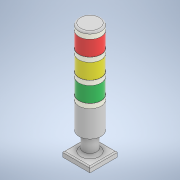
# Autodesk Inventor part: 警示燈
Saved by Autodesk Inventor 2022 (Build 260153000, 153)
## iProperties
Created: 2023-03-12
Part Number: 警示燈
Material: 一般
Document SubType Name: Modeling
Designer: User
Mass: 907.792 g
Surface Area: 752.97 cm^2
Volume: 907.792 cm^3
Density: 1 g/cm^3
Appearance: 預設
Author: User
Autodesk Inventor part; units mm, degrees
ref_plane "YZ Plane" through (0, 0, 0) normal (1, 0, 0) x (0, 1, 0)
ref_plane "XZ Plane" through (0, 0, 0) normal (0, 1, 0) x (-1, 0, 0)
ref_plane "XY Plane" through (0, 0, 0) normal (0, 0, 1) x (1, 0, 0)
sketch "草圖1" plane through (0, 0, 0) normal (0, 0, 1) x (1, 0, 0)
  line L0 (-6.2319, 0) -> (37.3914, 0) construction
  line L1 (0, -62.7215) -> (0, 388.8794) construction
  line L2 (0, 324.365) -> (31.1595, 324.365)
  line L3 (31.1595, 324.365) -> (31.1595, 65.285)
  line L4 (31.1595, 65.285) -> (0, 65.285)
  line L5 (0, 65.285) -> (0, 324.365)
  line L6 (0, 65.285) -> (18.4838, 65.285)
  line L7 (18.4838, 65.285) -> (18.4838, 1.7929)
  line L8 (18.4838, 1.7929) -> (0, 1.7929)
  line L9 (0, 1.7929) -> (0, 65.285)
  line L10 (31.1595, 306.585) -> (30.6515, 306.585)
  line L11 (30.6515, 306.585) -> (30.6515, 263.405)
  line L12 (30.6515, 263.405) -> (31.1595, 263.405)
  line L13 (31.1595, 263.405) -> (31.1595, 306.585)
  line L14 (31.1595, 250.705) -> (30.6515, 250.705)
  line L15 (30.6515, 250.705) -> (30.6515, 207.525)
  line L16 (30.6515, 207.525) -> (31.1595, 207.525)
  line L17 (31.1595, 207.525) -> (31.1595, 250.705)
  line L18 (31.1595, 194.825) -> (30.6515, 194.825)
  line L19 (30.6515, 194.825) -> (30.6515, 151.645)
  line L20 (30.6515, 151.645) -> (31.1595, 151.645)
  line L21 (31.1595, 151.645) -> (31.1595, 194.825)
  line L22 (31.1595, 138.945) -> (30.6515, 138.945)
  line L23 (30.6515, 138.945) -> (30.6515, 65.285)
  line L24 (30.6515, 65.285) -> (31.1595, 65.285)
  line L25 (31.1595, 65.285) -> (31.1595, 138.945)
  point P0 (31.1595, 151.645)
  point P1 (31.1595, 207.525)
  point P2 (31.1595, 263.405)
  dimension "d7" = 0.508
  dimension "d8" = 43.18
  dimension "d9" = 43.18
  dimension "d10" = 17.78
  dimension "d11" = 12.7
  dimension "d12" = 12.7
  dimension "d13" = 43.18
  dimension "d18" = 12.7
  constraints: 48 end point, 12 parallel, 8 point on line, 6 horizontal, 6 perpendicular, 1 midpoint
  measures "d7" distance of L10.start L10.end
  measures "d8" distance of L10.end L11.end
  measures "d9" distance of L14.end L15.end
  measures "d10" distance between parallel lines of L10 L2
  measures "d11" distance between parallel lines of L14 L12
  measures "d12" distance between parallel lines of L18 L16
  measures "d13" distance of L18.end L19.end
  measures "d18" distance between parallel lines of L22 L20
revolve "迴轉1" add sketch "草圖1" angle 360 about axis through (0, 65.285, 0) along (0, 1, 0)
sketch "草圖2" plane through (0, 0, 0) normal (0, 1, 0) x (-1, 0, 0)
  line L0 (38.1, -38.1) -> (-38.1, -38.1)
  line L1 (-38.1, -38.1) -> (-38.1, 38.1)
  line L2 (-38.1, 38.1) -> (38.1, 38.1)
  line L3 (38.1, 38.1) -> (38.1, -38.1)
  line L4 (53.34, 0) -> (-53.34, 0) construction
  line L5 (0, -53.34) -> (0, 53.34) construction
  point P0 (0, 0)
  dimension "d5" = 76.2
  dimension "d6" = 76.2
  constraints: 8 end point, 2 parallel, 1 horizontal, 1 perpendicular, 2 other
  measures "d5" distance of L0.start L0.end
  measures "d6" distance of L2.end L0.start
extrude "擠出1" add sketch "草圖2" along normal blind 14.2875
revolve "迴轉2" cut sketch "草圖1" angle 360 about axis through (0, -10, 0) along (0, 1, 0) contours L3 L12 L11 L10 | L23 L22 L3 L4 | L3 L16 L15 L14 | L3 L20 L19 L18
fillet "圓角1" radius 5.08 1 edges at (-31.1595, 324.365, 0)
fillet "圓角2" radius 7.62 1 edges at (-18.4838, 14.2875, 0)
fillet "圓角3" radius 3.175 4 edges at (38.1, 14.2875, 0) (-38.1, 14.2875, 0) (0, 14.2875, 38.1) (0, 14.2875, -38.1)
